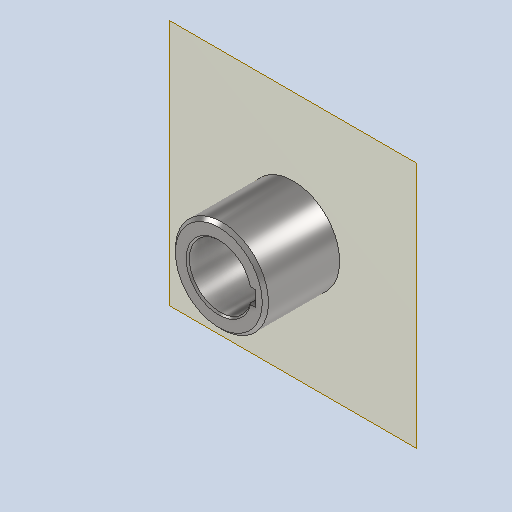
# Autodesk Inventor part: Część7
Saved by Autodesk Inventor 2024 (Build 280153000, 153)
## iProperties
Created: 2023-11-21
Part Number: Część7
Material: Stal nierdzewna
Document SubType Name: Modeling
Designer: Wojciech
Density: 8 g/cm^3
Appearance: Częściowo polerowany
Author: Wojciech
Autodesk Inventor part; units mm, degrees
ref_plane "YZ Plane" through (0, 0, 0) normal (1, 0, 0) x (0, 1, 0)
ref_plane "XZ Plane" through (0, 0, 0) normal (0, 1, 0) x (-1, 0, 0)
ref_plane "XY Plane" through (0, 0, 0) normal (0, 0, 1) x (1, 0, 0)
ref_plane "Płaszczyzna konstrukcyjna1" through (0, 0, 0) normal (0, 0, 1) x (1, 0, 0)
sketch "Szkic1" plane through (0, 0, 0) normal (0, 0, 1) x (1, 0, 0)
  arc A0 (19.3649, 5) -> (19.3649, -5) centre (0, 0) ccw projected
  line L0 (19.3649, 5) -> (24, 5) projected
  line L1 (24, 5) -> (24, -5) projected
  line L2 (24, -5) -> (19.3649, -5) projected
  circle A1 centre (0, 0) radius 30
  dimension "d0" = 60
  constraints: 1 centre point, 1 coincident, 2 other
  measures "d0" diameter of A1
extrude "Wyciągnięcie proste1" add sketch "Szkic1" along normal blind 48
chamfer "Faza1" distance 2 angle 45 1 edges at (-30, 0, 48)
chamfer "Faza2" distance 1 angle 45 1 edges at (-20, 0, 48)
